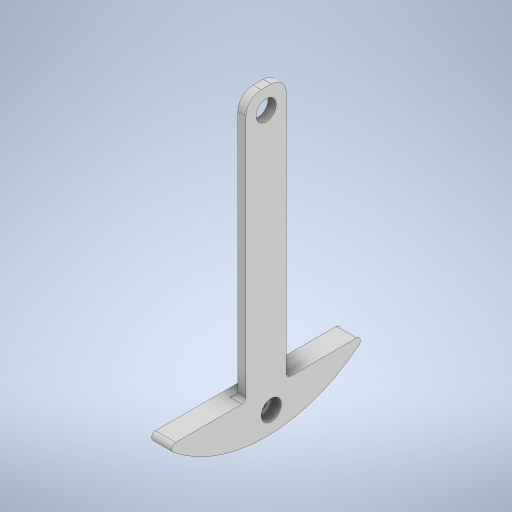
# Autodesk Inventor part: 受動歩行_ver3
Saved by Autodesk Inventor 2023 (Build 270158000, 158)
## iProperties
Created: 2024-05-31
Part Number: 受動歩行_ver3
Material: 一般
Document SubType Name: Modeling
Designer: babar
Density: 1 g/cm^3
Appearance: 既定
Author: babar
Autodesk Inventor part; units mm, degrees
ref_plane "YZ Plane" through (0, 0, 0) normal (1, 0, 0) x (0, 1, 0)
ref_plane "XZ Plane" through (0, 0, 0) normal (0, 1, 0) x (-1, 0, 0)
ref_plane "XY Plane" through (0, 0, 0) normal (0, 0, 1) x (1, 0, 0)
sketch "スケッチ4" plane through (0, 0, 0) normal (1, 0, 0) x (0, 1, 0)
  line L0 (0, 0) -> (0, -100)
  line L1 (0, -50) -> (-20, -50)
  arc A0 (0, 0) -> (0, -100) centre (52.5, -50) ccw
  dimension "d23" = 100
  dimension "d24" = 20
  constraints: 4 end point, 3 point on circle, 1 centre point, 1 horizontal, 1 midpoint, 1 vertical
  measures "d23" distance of L0.start L0.end
  measures "d24" distance of L1.start L1.end
extrude "押し出し3" add sketch "スケッチ4" against normal blind 10
sketch "スケッチ5" plane through (0, 0, 0) normal (1, 0, 0) x (0, 0, -1)
  line L0 (40, 130) -> (60, 130)
  line L1 (60, 130) -> (60, 0)
  line L2 (60, 0) -> (40, 0)
  line L3 (40, 0) -> (40, 130)
  line L4 (100, 0) -> (0, 0) projected
  point P0 (50, 0)
  point P1 (50, 0)
  dimension "d27" = 20
  dimension "d28" = 130
  dimension "d29" = 0
  dimension "d30" = 0
  constraints: 8 end point, 2 midpoint, 2 parallel, 1 horizontal, 1 perpendicular
  measures "d27" distance of L0.start L0.end
  measures "d28" distance of L0.end L1.end
  measures "d29" distance between parallel lines of L4 L2
  measures "d30" distance of point (50, 0) point (50, 0)
extrude "押し出し4" add sketch "スケッチ5" against normal blind 4
sketch "スケッチ6" plane through (0, 0, 0) normal (1, 0, 0) x (0, 0, -1)
  line L0 (60, 0) -> (60, 130) projected
  line L1 (60, 130) -> (40, 130) projected
  point P0 (0, 0)
  point P1 (50, 120)
  dimension "d33" = 10
  dimension "d34" = 10
  measures "d33" distance from line of L0 point (50, 120)
  measures "d34" distance from line of L1 point (50, 120)
hole "穴2" at (0, 120, -50) direction (-1, 0, 0) diameter 10 end through all
sketch "スケッチ7" plane through (0, 0, 0) normal (1, 0, 0) x (0, 0, -1)
  line L0 (40, 0) -> (60, 0) projected
  line L1 (60, 0) -> (60, 130) projected
  point P0 (0, 0)
  point P1 (52.5, -9.6825)
  point P2 (50, 0)
  dimension "d42" = 10
  dimension "d43" = 7.5
  constraints: 1 midpoint
  measures "d42" distance of point (50, 0) point (52.5, -9.682)
  measures "d43" distance from line of L1 point (52.5, -9.682)
hole "穴3" at (0, -9.6825, -52.5) direction (-1, 0, 0) diameter 6 end through all counterbore diameter 10 counterbore depth 5
fillet "フィレット1" radius 7.5 2 edges at (-2, 130, -40) (-2, 130, -60)
fillet "フィレット2" radius 2 3 edges at (-2, 0, -40) (-4, 0, -50) (-2, 0, -60)
fillet "フィレット3" radius 2 2 edges at (-5, 0, 0) (-5, 0, -100)
